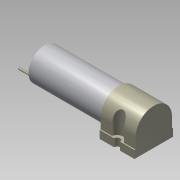
# Autodesk Inventor part: valve
Saved by Autodesk Inventor 2014 (Build 180170000, 170)
## iProperties
Created: 2013-10-04
Part Number: valve
Material: PVC-Piping
Document SubType Name: Modeling
Designer: Admin
Density: 1 g/cm^3
Appearance: Smooth - White(3)
Author: Admin
Autodesk Inventor part; units mm, degrees
ref_plane "YZ Plane" through (0, 0, 0) normal (1, 0, 0) x (0, 1, 0)
ref_plane "XZ Plane" through (0, 0, 0) normal (0, 1, 0) x (-1, 0, 0)
ref_plane "XY Plane" through (0, 0, 0) normal (0, 0, 1) x (1, 0, 0)
sketch "Sketch5" plane through (0, 0, 0) normal (0, 0, 1) x (1, 0, 0)
  line L0 (4.757, -5.8274) -> (-6.673, -5.8274)
  line L1 (-6.673, -5.8274) -> (-6.673, 6.8226)
  line L2 (-6.673, 6.8226) -> (4.757, 6.8226)
  line L3 (4.757, 6.8226) -> (4.757, -5.8274)
  circle A0 centre (-0.958, 0.4976) radius 0.76
  circle A1 centre (2.222, 0.4976) radius 0.76
  circle A2 centre (-4.138, 0.4976) radius 0.76
  point P0 (0, 0)
  dimension "d15" = 11.43
  dimension "d16" = 12.65
  dimension "d17" = 1.52
  dimension "d18" = 1.52
  dimension "d19" = 1.52
  dimension "d20" = 3.18
  dimension "d21" = 3.18
  constraints: 8 end point, 3 centre point, 2 parallel, 1 horizontal, 1 perpendicular
  measures "d15" distance of L1.end L2.end
  measures "d16" distance of L0.end L1.end
  measures "d17" diameter of A0
  measures "d18" diameter of A1
  measures "d19" diameter of A2
  measures "d20" distance of A1.centre A0.centre
  measures "d21" distance of A0.centre A2.centre
extrude "Extrusion4" add sketch "Sketch5" along normal blind 2.54
sketch "Sketch6" plane through (0, 0, 2.54) normal (0, 0, 1) x (1, 0, 0)
  line L0 (4.757, 6.8226) -> (-6.673, 6.8226) projected
  circle A0 centre (-0.958, 6.8226) radius 1
  point P0 (0, 0)
  dimension "d24" = 2
  constraints: 1 centre point, 1 midpoint
  measures "d24" diameter of A0
extrude "Extrusion5" cut sketch "Sketch6" against normal blind 2.54
sketch "Sketch7" plane through (0, 0, 2.54) normal (0, 0, 1) x (1, 0, 0)
  line L0 (-6.673, -5.8274) -> (4.757, -5.8274) projected
  circle A0 centre (-0.958, -5.8274) radius 1
  point P0 (0, 0)
  dimension "d27" = 2
  constraints: 1 centre point, 1 midpoint
  measures "d27" diameter of A0
extrude "Extrusion6" cut sketch "Sketch7" against normal blind 2.54
move or copy body "Move Body1" bodies to move or copy 1 copy no translate (1, -0.5, 0)
sketch "Sketch14" plane through (-5.673, -6.3274, 0) normal (-1, 0, 0) x (0, 0, 1)
  arc A0 (5.97, 0.3574) -> (5.97, 12.2974) centre (5.97, 6.3274) ccw
  line L0 (5.97, 12.2974) -> (5.97, 0.3574)
  dimension "d37" = 5.97
  constraints: 2 end point, 2 point on circle, 1 centre point, 1 vertical
  measures "d37" radius of A0
extrude "Extrusion7" add sketch "Sketch14" against normal blind 11.43
sketch "Sketch15" plane through (-5.673, -5.97, 5.97) normal (0, 0, -1) x (-1, 0, 0)
  line L0 (0, 11.94) -> (-11.43, 11.94)
  line L1 (-11.43, 11.94) -> (-11.43, 0)
  line L2 (-11.43, 0) -> (0, 0)
  line L3 (0, 0) -> (0, 11.94)
  point P0 (-5.673, 5.97)
  constraints: 8 end point, 2 parallel, 1 horizontal, 1 perpendicular
extrude "Extrusion8" add sketch "Sketch15" along normal blind 3.43
sketch "Sketch16" plane through (-5.673, 6.3226, 2.54) normal (0, 0, 1) x (1, 0, 0)
  arc A0 (4.715, 0) -> (4.7792, -0.3526) centre (5.715, 0) ccw projected
  circle A1 centre (5.715, 0) radius 2
  point P0 (5.673, -6.3226)
  dimension "d42" = 4
  constraints: 1 centre point, 1 coincident
  measures "d42" diameter of A1
extrude "Extrusion9" cut sketch "Sketch16" along normal blind 9.68
sketch "Sketch17" plane through (-5.673, -6.3274, 2.54) normal (0, 0, 1) x (1, 0, 0)
  arc A0 (4.781, 0.3574) -> (4.715, 0) centre (5.715, 0) ccw projected
  circle A1 centre (5.715, 0) radius 2
  point P0 (5.673, 6.3274)
  dimension "d45" = 4
  constraints: 1 centre point, 1 coincident
  measures "d45" diameter of A1
extrude "Extrusion10" cut sketch "Sketch17" along normal blind 9.68
sketch "Sketch18" plane through (-5.673, -6.3274, 0) normal (-1, 0, 0) x (0, 0, 1)
  arc A0 (5.97, 0.3574) -> (5.97, 12.2974) centre (5.97, 6.3274) ccw projected
  circle A1 centre (5.97, 6.3274) radius 5.2674
  point P0 (0, 6.3274)
  constraints: 1 centre point, 1 coincident
extrude "Extrusion11" add sketch "Sketch18" along normal blind 24.38
sketch "Sketch20" plane through (-30.053, 0, 5.97) normal (-1, 0, 0) x (0, 0, 1)
  circle A0 centre (0, 0) radius 5.2674 projected
  circle A1 centre (-3, 2.5) radius 0.35
  line L0 (-10.3331, 0) -> (11.6228, 0)
  circle A2 centre (-3, -2.5) radius 0.35
  point P0 (-5.97, 0)
  dimension "d50" = 2.5
  dimension "d51" = 3
  dimension "d52" = 0.7
  constraints: 2 centre point, 2 end point, 1 horizontal, 1 symmetric about line, 1 other
  measures "d50" vertical distance of A0.centre A1.centre
  measures "d51" horizontal distance of A0.centre A1.centre
  measures "d52" diameter of A1
extrude "Extrusion12" add sketch "Sketch20" along normal blind 6 contours A1 | A2
fillet "Fillet1" radius 0.2 4 edges at (-30.053, -2.5, 2.62) (-30.053, 2.5, 2.62) (-36.053, 2.5, 2.62) (-36.053, -2.5, 2.62)
body "Solid2"
